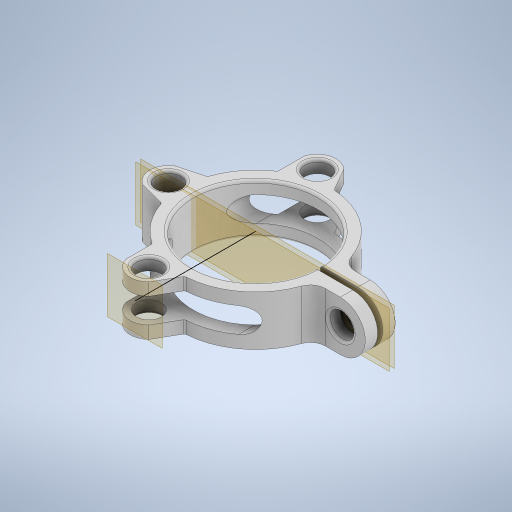
# Autodesk Inventor part: 19th_choibeomsu_01
Saved by Autodesk Inventor 2024 (Build 280153000, 153)
## iProperties
Created: 2024-08-06
Part Number: 19th_choibeomsu_01
Material: 일반
Document SubType Name: Modeling
Designer: chlqj
Density: 1 g/cm^3
Appearance: 기본값
Author: chlqj
Autodesk Inventor part; units mm, degrees
ref_plane "YZ Plane" through (0, 0, 0) normal (1, 0, 0) x (0, 1, 0)
ref_plane "XZ Plane" through (0, 0, 0) normal (0, 1, 0) x (-1, 0, 0)
ref_plane "XY Plane" through (0, 0, 0) normal (0, 0, 1) x (1, 0, 0)
sketch "스케치1" plane through (0, 0, 0) normal (0, 1, 0) x (-1, 0, 0)
  line L0 (0, 0) -> (35, 0) construction
  line L1 (0, 0) -> (80, 0) construction
  circle A0 centre (9.0587, -33.8074) radius 5
  circle A1 centre (9.0587, 33.8074) radius 5
  line L2 (0, 0) -> (35, 0)
  circle A2 centre (35, 0) radius 5
  line L3 (35, 7.5) -> (29.0647, 9.0903)
  line L4 (35, 7.5) -> (41.1446, 7.5) construction
  line L5 (35, -7.5) -> (29.0647, -9.0903)
  line L6 (35, -7.5) -> (41.1446, -7.5) construction
  line L7 (35, 7.5) -> (38.75, 6.4952)
  line L8 (35, -7.5) -> (38.75, -6.4952)
  arc A3 (38.75, -6.4952) -> (38.75, 6.4952) centre (35, 0) ccw
  line L9 (9.0587, 33.8074) -> (15.6639, 58.4585)
  line L10 (9.0587, 33.8074) -> (34.5793, 33.8074) construction
  line L11 (16.3031, 31.8663) -> (16.3031, 25.7216)
  line L12 (16.3031, 31.8663) -> (38.5294, 31.8663) construction
  arc A4 (16.3031, 35.7485) -> (3.7554, 39.1107) centre (9.0587, 33.8074) ccw
  line L13 (3.7554, 39.1107) -> (-1.2581, 30.4271)
  line L14 (16.3031, 35.7485) -> (16.3031, 25.1835)
  line L15 (1.8142, -35.7485) -> (7.7668, -35.7485) construction
  arc A5 (3.7554, -39.1107) -> (16.3031, -35.7485) centre (9.0587, -33.8074) ccw
  line L16 (16.3031, -25.7216) -> (16.3031, -35.7485)
  line L17 (-1.2581, -30.4271) -> (3.7554, -39.1107)
  arc A6 (3.7554, -39.1107) -> (16.3031, -35.7485) centre (9.0587, -33.8074) ccw
  arc A7 (16.7449, -24.8919) -> (28.3776, -9.7319) centre (0, 0) ccw
  arc A8 (28.3776, 9.7319) -> (16.7449, 24.8919) centre (0, 0) ccw
  arc A9 (16.7449, -24.8919) -> (16.3031, -25.7216) centre (17.3031, -25.7216) ccw
  arc A10 (29.0647, -9.0903) -> (28.3776, -9.7319) centre (29.3236, -10.0563) ccw
  arc A11 (16.3031, 25.7216) -> (16.7449, 24.8919) centre (17.3031, 25.7216) ccw
  arc A12 (28.3776, 9.7319) -> (29.0647, 9.0903) centre (29.3236, 10.0563) ccw
  arc A13 (-2.0556, 29.9295) -> (-1.2581, 30.4271) centre (-2.1241, 30.9271) ccw
  arc A14 (-1.2581, -30.4271) -> (-2.0556, -29.9295) centre (-2.1241, -30.9271) ccw
  line L18 (0, -48.9967) -> (-40, -48.9967)
  line L19 (0, -59.9761) -> (-50, -59.9761)
  line L20 (-40, -1) -> (-50, -1)
  line L21 (-40, 1) -> (-50, 1)
  line L22 (-50, -1) -> (-50, -6)
  line L23 (-50, 1) -> (-50, 6)
  line L24 (-50, 6) -> (-33.9411, 6)
  line L25 (-50, -6) -> (-33.9411, -6)
  line L26 (-50, -1) -> (-24.98, -1)
  line L27 (-50, 1) -> (-24.98, 1)
  arc A15 (-2.0556, 29.9295) -> (-28.2843, 10) centre (0, 0) ccw
  arc A16 (-28.2843, -10) -> (-2.0556, -29.9295) centre (0, 0) ccw
  arc A17 (-24.98, -1) -> (-24.98, 1) centre (0, 0) ccw
  arc A18 (-30.1993, 6) -> (-29.2252, 6.7742) centre (-30.1993, 7) ccw
  arc A19 (-33.9411, 6) -> (-28.2843, 10) centre (-33.9411, 12) ccw
  arc A20 (-28.2843, -10) -> (-33.9411, -6) centre (-33.9411, -12) ccw
  point P0 (28.5449, 9.2296)
  point P1 (28.5449, -9.2296)
  point P2 (-1.5272, 29.9611)
  point P3 (16.3031, -25.1835)
  point P4 (-1.5272, -29.9611)
  point P5 (-29.3939, 6)
  point P6 (-29.3939, -6)
  dimension "d12" = 35
  dimension "d15" = 165
  dimension "d16" = 165
  dimension "d18" = 75
  dimension "d23" = 1
  dimension "d24" = 1
  dimension "d25" = 1
  dimension "d26" = 1
  dimension "d28" = 10
  dimension "d29" = 10
  dimension "d30" = 10
  dimension "d31" = 40
  dimension "d32" = 50
  dimension "d35" = 5
  dimension "d36" = 5
  constraints: 56 end point, 43 point on circle, 21 centre point, 16 tangent, 11 horizontal, 10 point on line, 7 vertical, 3 equal length, 3 equal radius, 2 coincident, 2 collinear, 1 parallel, 1 perpendicular, 4 other
  measures "d12" distance of L0.start L0.end
  measures "d15" angle of L4 L3
  measures "d16" angle of L5 L6
  measures "d18" angle of L10 L9
  measures "d23" radius of A9
  measures "d24" radius of A10
  measures "d25" radius of A11
  measures "d26" radius of A13
  measures "d28" diameter of A0
  measures "d29" diameter of A2
  measures "d30" diameter of A1
  measures "d31" distance of L18.start L18.end
  measures "d32" distance of L19.start L19.end
  measures "d35" distance of L20.end L22.end
  measures "d36" distance of L21.end L23.end
extrude "돌출1" add sketch "스케치1" along normal blind 20
fillet "모깎기1" radius 1 3 edges at (-4.0587, 20, 33.8074) (-30, 20, 0) (-4.0587, 20, -33.8074)
fillet "모깎기2" radius 10 1 edges at (50, 20, -3.5)
fillet "모깎기3" radius 10 3 edges at (50, 0, -3.5) (50, 0, 3.5) (50, 20, 3.5)
ref_plane "작업 평면2" through (32.49, 20, -1) normal (0, 0, 1) x (-1, 0, 0)
ref_plane "작업 평면1" through (50, 20, 1) normal (0, 0, 1) x (-1, 0, 0)
fillet "모깎기4" radius 1 3 edges at (-4.0587, 0, 33.8074) (-30, 0, 0) (-4.0587, 0, -33.8074)
sketch "스케치2" plane through (0, 20, 0) normal (0, 1, 0) x (1, 0, 0)
  line L0 (0, 0) -> (0, -48.5366)
  constraints: 2 end point, 1 vertical
ref_plane "작업 평면3" through (0, 20, 48.5366) normal (0, 0, 1) x (1, 0, 0)
sketch "스케치3" plane through (0, 20, 48.5366) normal (0, 0, 1) x (1, 0, 0)
  line L0 (0, -20) -> (0, -15)
  line L1 (-17.51, -15) -> (17.49, -15)
  line L2 (17.49, -5) -> (-17.51, -5)
  line L3 (-17.51, -15) -> (17.49, -5) construction
  line L4 (17.49, -15) -> (-17.51, -5) construction
  arc A0 (14.8485, -14.2453) -> (14.8485, -5.7547) centre (17.49, -10) ccw
  arc A1 (-14.8685, -5.7547) -> (-14.8685, -14.2453) centre (-17.51, -10) ccw
  point P0 (-0.01, -10)
  dimension "d46" = 5
  dimension "d47" = 35
  dimension "d48" = 10
  dimension "d49" = 10
  dimension "d50" = 10
  constraints: 10 end point, 4 point on circle, 4 point on line, 2 centre point, 2 midpoint, 1 horizontal, 1 parallel, 1 vertical
  measures "d46" distance of L0.start L0.end
  measures "d47" distance of L2.end L2.start
  measures "d48" distance of L2.start L1.end
  measures "d49" diameter of A0
  measures "d50" diameter of A1
extrude "돌출2" cut sketch "스케치3" against normal blind 200
sketch "스케치4" plane through (33.9411, 0, 6) normal (0, 0, 1) x (1, 0, 0)
  arc A0 (6.0589, 0) -> (6.0589, 20) centre (6.0589, 10) ccw projected
  line L0 (6.0589, 20) -> (6.0589, 0)
  circle A1 centre (6.0589, 10) radius 5
  point P0 (-33.9411, 0)
  dimension "d53" = 10
  constraints: 2 end point, 1 centre point, 1 coincident, 1 vertical
  measures "d53" diameter of A1
extrude "돌출3" cut sketch "스케치4" against normal blind 200 contours A1 L0 | L0 A1
fillet "모깎기5" radius 1 4 edges at (35, 10, 6) (35, 10, -6) (-25, 20, 0) (-25, 0, 0)
